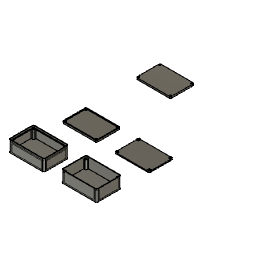
Customizable_project_box_v2_v3 (Autodesk Fusion 360 design; units mm, degrees)
Autodesk Fusion 360 part; units mm, degrees
sketch "Box footprint" plane through (0, 0, 0) normal (0, 0, 1) x (1, 0, 0)
  line L0 (0, 0) -> (130, 0)
  line L1 (130, 0) -> (130, 90)
  line L2 (130, 90) -> (0, 90)
  line L3 (0, 90) -> (0, 0)
  circle A0 centre (125.5, 85.5) radius 1.35
  line L4 (130, 90) -> (121, 90)
  line L5 (121, 90) -> (121, 81)
  line L6 (121, 81) -> (130, 81)
  line L7 (130, 81) -> (130, 90)
  line L8 (0, 81) -> (9, 81)
  line L9 (0, 90) -> (0, 81)
  line L10 (9, 81) -> (9, 90)
  line L11 (9, 90) -> (0, 90)
  circle A1 centre (4.5, 85.5) radius 1.35
  line L12 (121, 0) -> (130, 0)
  line L13 (121, 9) -> (121, 0)
  line L14 (130, 0) -> (130, 9)
  line L15 (130, 9) -> (121, 9)
  circle A2 centre (125.5, 4.5) radius 1.35
  line L16 (0, 0) -> (9, 0)
  line L17 (0, 9) -> (0, 0)
  line L18 (9, 0) -> (9, 9)
  line L19 (9, 9) -> (0, 9)
  circle A3 centre (4.5, 4.5) radius 1.35
  line L20 (4, 4) -> (126, 4) construction
  line L21 (126, 4) -> (126, 86) construction
  line L22 (126, 86) -> (4, 86) construction
  line L23 (4, 86) -> (4, 4) construction
  arc A4 (0, 4) -> (4, 0) centre (4, 4) ccw
  arc A5 (4, 90) -> (0, 86) centre (4, 86) ccw
  arc A6 (130, 86) -> (126, 90) centre (126, 86) ccw
  arc A7 (126, 0) -> (130, 4) centre (126, 4) ccw
  point P0 (125.5, 85.5)
  dimension "d1" = 130
  dimension "d2" = 90
  dimension "d13" = 2.7
  dimension "d14" = 9
  dimension "d15" = 9
  dimension "d19" = 2.7
  dimension "d20" = 9
  dimension "d21" = 9
  dimension "d22" = 2.7
  dimension "d23" = 9
  dimension "d24" = 9
  dimension "d28" = 2.7
  dimension "d29" = 9
  dimension "d30" = 9
  dimension "d125" = 4.5
  dimension "d126" = 4.5
  dimension "d127" = 4.5
  dimension "d128" = 4.5
  dimension "d177" = 4
  dimension "d178" = 4
  dimension "d179" = 4
  dimension "d180" = 4
  constraint horizontal L0
  constraint vertical L1
  constraint horizontal L2
  constraint vertical L3
  constraint coincident L0.start L3.end
  constraint horizontal L4
  constraint perpendicular L4 L5
  constraint parallel L4 L6
  constraint parallel L5 L7
  constraint coincident P0 A0.centre
  constraint horizontal L11
  constraint perpendicular L9 L11
  constraint parallel L8 L11
  constraint parallel L9 L10
  constraint horizontal L15
  constraint perpendicular L13 L15
  constraint parallel L12 L15
  constraint parallel L13 L14
  constraint horizontal L19
  constraint perpendicular L17 L19
  constraint parallel L16 L19
  constraint parallel L17 L18
  constraint coincident L2.end L3.start
  constraint coincident L0.end L1.start
  constraint vertical A1.centre A3.centre
  constraint vertical P0 A2.centre
  constraint horizontal P0 A1.centre
  constraint horizontal A2.centre A3.centre
  constraint horizontal L20
  constraint vertical L21
  constraint horizontal L22
  constraint vertical L23
  constraint coincident L17 A4.start
  constraint coincident L20.start L23.end
  constraint horizontal L20.start A4.start
  constraint vertical L20.start A4.end
  constraint coincident L9 A5.end
  constraint coincident L22.end L23.start
  constraint horizontal L22.end A5.end
  constraint vertical L22.end A5.start
  constraint coincident L4 A6.end
  constraint coincident L21.end L22.start
  constraint vertical L21.end A6.end
  constraint horizontal L21.end A6.start
  constraint coincident L12 A7.start
  constraint coincident L20.end L21.start
  constraint vertical L20.end A7.start
  constraint horizontal L20.end A7.end
  measures "d1" distance of L0.start L0.end
  measures "d2" distance of L0.start L2.end
  measures "d13" diameter of A0
  measures "d14" distance of L5.end L6.end
  measures "d15" distance of L4.end L5.end
  measures "d19" diameter of A1
  measures "d20" distance of L8.start L8.end
  measures "d21" distance of L2.end L8.start
  measures "d22" diameter of A2
  measures "d23" distance of L12.start L0.end
  measures "d24" distance of L13.start L12.start
  measures "d28" diameter of A3
  measures "d29" distance of L0.start L16.end
  measures "d30" distance of L17.start L0.start
  measures "d125" distance of A1.centre L9
  measures "d126" distance of L1 P0
  measures "d127" distance of L0 A2.centre
  measures "d128" distance of L2 P0
  measures "d177" distance of L0 L20
  measures "d178" distance of L3 L23
  measures "d179" distance of L1 L21
  measures "d180" distance of L2 L22
extrude "Extrude1" add sketch "Box footprint" against normal blind 4 contours L0 L3 L16 L17 L18 L19 A4 | L0 L1 L2 L3 L5 L6 L8 L10 L13 L15 L18 L19 | L0 L1 L12 L13 L14 L15 A7 | L2 L3 L8 L9 L10 L11 A5 | L1 L2 L4 L5 L6 L7 A6 | A0 | A1 | A2 | A3 makes body 1
extrude "Extrude5" add sketch "Box footprint" along normal blind 2 contours L0 L3 L16 L17 L18 L19 A4 | L0 L1 L12 L13 L14 L15 A7 | L2 L3 L8 L9 L10 L11 A5 | L1 L2 L4 L5 L6 L7 A6 | A0 | A1 | A2 | A3 bodies 1
sketch "Lid outline" plane through (0, 0, -4) normal (0, 0, -1) x (1, 0, 0)
  arc A0 (4, 0) -> (0, -4) centre (4, -4) ccw
  arc A1 (0, -86) -> (4, -90) centre (4, -86) ccw
  arc A2 (126, -90) -> (130, -86) centre (126, -86) ccw
  arc A3 (130, -4) -> (126, 0) centre (126, -4) ccw
  line L0 (126, 0) -> (4, 0)
  line L1 (0, -4) -> (0, -86)
  line L2 (4, -90) -> (126, -90)
  line L3 (130, -86) -> (130, -4)
  line L4 (-0.2, -4) -> (-0.2, -86)
  arc A4 (-0.2, -86) -> (4, -90.2) centre (4, -86) ccw
  line L5 (4, -90.2) -> (126, -90.2)
  arc A5 (126, -90.2) -> (130.2, -86) centre (126, -86) ccw
  line L6 (130.2, -86) -> (130.2, -4)
  arc A6 (130.2, -4) -> (126, 0.2) centre (126, -4) ccw
  line L7 (126, 0.2) -> (4, 0.2)
  arc A7 (4, 0.2) -> (-0.2, -4) centre (4, -4) ccw
  line L8 (126, 2) -> (4, 2)
  arc A8 (4, 2) -> (-2, -4) centre (4, -4) ccw
  line L9 (-2, -4) -> (-2, -86)
  arc A9 (-2, -86) -> (4, -92) centre (4, -86) ccw
  line L10 (4, -92) -> (126, -92)
  arc A10 (126, -92) -> (132, -86) centre (126, -86) ccw
  line L11 (132, -86) -> (132, -4)
  arc A11 (132, -4) -> (126, 2) centre (126, -4) ccw
  line L12 (121, -9) -> (121, 0.2)
  line L13 (121, -9) -> (130.2, -9)
  line L14 (121, -81) -> (121, -90.2)
  line L15 (121, -81) -> (130.2, -81)
  line L16 (9, -81) -> (9, -90.2)
  line L17 (9, -81) -> (-0.2, -81)
  line L18 (9, -9) -> (-0.2, -9)
  line L19 (9, -9) -> (9, 0.2)
  circle A12 centre (4.5, -85.5) radius 1.35
  circle A13 centre (4.5, -4.5) radius 1.35
  circle A14 centre (125.5, -4.5) radius 1.35
  circle A15 centre (125.5, -85.5) radius 1.35
  point P0 (9, -9)
  point P1 (9, -81)
  point P2 (121, -81)
  point P3 (121, -9)
  dimension "d181" = 0.2
  dimension "d182" = 2
  constraint coincident A3.end L0.start
  constraint coincident A0.start L0.end
  constraint coincident A0.end L1.start
  constraint coincident A1.start L1.end
  constraint coincident A1.end L2.start
  constraint coincident A2.start L2.end
  constraint coincident A2.end L3.start
  constraint coincident A3.start L3.end
  constraint coincident P3 L12.start
  constraint coincident L7 L12.end
  constraint perpendicular L7 L12
  constraint coincident L6 L13.end
  constraint perpendicular L6 L13
  constraint coincident P2 L14.start
  constraint coincident L5 L14.end
  constraint perpendicular L5 L14
  constraint coincident L6 L15.end
  constraint perpendicular L6 L15
  constraint coincident P1 L16.start
  constraint coincident L5 L16.end
  constraint perpendicular L5 L16
  constraint coincident L4 L17.end
  constraint perpendicular L4 L17
  constraint coincident P0 L18.start
  constraint coincident L4 L18.end
  constraint perpendicular L4 L18
  constraint coincident L7 L19.end
  constraint perpendicular L7 L19
extrude "Extrude8" add sketch "Lid outline" against normal blind 39 separate body contours L8 A8 L9 A9 L10 A10 L11 A11 makes body 2
sketch "Lid screw holes" plane through (0, 0, 35) normal (0, 0, 1) x (-1, 0, 0)
  circle A0 centre (-4.5, -85.5) radius 1.7
  circle A1 centre (-4.5, -4.5) radius 1.7
  circle A2 centre (-125.5, -4.5) radius 1.7
  circle A3 centre (-125.5, -85.5) radius 1.7
  circle A4 centre (-125.5, -85.5) radius 3
  circle A5 centre (-125.5, -4.5) radius 3
  circle A6 centre (-4.5, -4.5) radius 3
  circle A7 centre (-4.5, -85.5) radius 3
  arc A8 (0.2, -4) -> (-4, 0.2) centre (-4, -4) ccw
  line L0 (0.2, -4) -> (0.2, -86)
  arc A9 (-4, -90.2) -> (0.2, -86) centre (-4, -86) ccw
  line L1 (-4, -90.2) -> (-126, -90.2)
  arc A10 (-130.2, -86) -> (-126, -90.2) centre (-126, -86) ccw
  line L2 (-130.2, -86) -> (-130.2, -4)
  arc A11 (-126, 0.2) -> (-130.2, -4) centre (-126, -4) ccw
  line L3 (-126, 0.2) -> (-4, 0.2)
  arc A12 (-126, 2) -> (-132, -4) centre (-126, -4) ccw
  line L4 (-132, -4) -> (-132, -86)
  arc A13 (-132, -86) -> (-126, -92) centre (-126, -86) ccw
  line L5 (-126, -92) -> (-4, -92)
  arc A14 (-4, -92) -> (2, -86) centre (-4, -86) ccw
  line L6 (2, -86) -> (2, -4)
  arc A15 (2, -4) -> (-4, 2) centre (-4, -4) ccw
  line L7 (-4, 2) -> (-126, 2)
  point P0 (-4.5, -85.5)
  point P1 (-4.5, -4.5)
  point P2 (-125.5, -4.5)
  point P3 (-125.5, -85.5)
  point P4 (-4, -76)
  point P5 (-4, -76)
  dimension "d63" = 3.4
  dimension "d64" = 3.4
  dimension "d65" = 3.4
  dimension "d66" = 3.4
  dimension "d67" = 6
  dimension "d68" = 6
  dimension "d69" = 6
  dimension "d70" = 6
  constraint coincident P1 A1.centre
  constraint concentric A3 A4
  constraint concentric A2 A5
  constraint concentric A1 A6
  constraint concentric A0 A7
  constraint coincident P0 A0.centre
  constraint coincident P2 A2.centre
  constraint coincident P3 A3.centre
  measures "d63" diameter of A0
  measures "d64" diameter of A1
  measures "d65" diameter of A2
  measures "d66" diameter of A3
  measures "d67" diameter of A4
  measures "d68" diameter of A5
  measures "d69" diameter of A6
  measures "d70" diameter of A7
extrude "Extrude9" add sketch "Lid screw holes" along normal blind 4 contours A0 | A1 | A2 | A3 | A4 | A5 | A6 | A7 | A8 L0 A9 L1 A10 L2 A11 L3 | A12 L4 A13 L5 A14 L6 A15 L7 bodies 2
extrude "Extrude16" add sketch "Lid outline" against normal up to surface (33 mm away) from surface at -6 contours A0 L0 L1 L18 L19 | A0 L0 L1 L4 L7 A7 L18 L19 | A3 L0 L3 L6 A6 L7 L12 L13 | A3 L0 L3 L12 L13 | A1 L1 L2 L16 L17 | A1 L1 L2 L4 A4 L5 L16 L17 | A2 L2 L3 L5 A5 L6 L14 L15 | A2 L2 L3 L14 L15 | A12 | A13 | A14 | A15 bodies 2
extrude "Extrude17" cut sketch "Lid outline" against normal blind 12 from surface at -6 contours A12 | A13 | A14 | A15 bodies 2
chamfer "Chamfer3" distance 0.8 angle 45 4 edges at (3.2414, 4.0118, 2) (124.2414, 4.0118, 2) (124.2414, 85.0118, 2) (3.2414, 85.0118, 2) on bodies 2
extrude "Extrude18" cut sketch "Lid screw holes" against normal up to surface (6 mm away) from surface at -33 contours A0 | A1 | A2 | A3 bodies 1
extrude "Extrude19" cut sketch "Lid screw holes" along normal blind 4 from surface at -39 contours A4 | A5 | A6 | A7 bodies 1
extrude "Extrude20" add sketch "Lid screw holes" along normal blind 0.2 from surface at -35 contours A0 | A1 | A2 | A3 bodies 1
sketch "Lid rebate" plane through (0, 0, 35) normal (0, 0, -1) x (1, 0, 0)
  line L0 (121, -2.8) -> (9, -2.8)
  line L1 (9, -87.2) -> (121, -87.2)
  line L2 (2.8, -9) -> (2.8, -81)
  line L3 (127.2, -81) -> (127.2, -9)
  line L4 (9, -81) -> (9, -90.2)
  line L5 (9, -81) -> (-0.2, -81)
  line L6 (4, -90.2) -> (126, -90.2)
  line L7 (-0.2, -4) -> (-0.2, -86)
  line L8 (9, -9) -> (-0.2, -9)
  line L9 (9, -9) -> (9, 0.2)
  line L10 (126, 0.2) -> (4, 0.2)
  line L11 (121, -9) -> (121, 0.2)
  line L12 (121, -9) -> (130.2, -9)
  line L13 (130.2, -86) -> (130.2, -4)
  line L14 (121, -81) -> (121, -90.2)
  line L15 (121, -81) -> (130.2, -81)
  dimension "d189" = 3
  dimension "d190" = 3
  dimension "d191" = 3
  dimension "d192" = 3
  constraint coincident L0.start L11
  constraint coincident L0.end L9
  constraint coincident L2.start L8
  constraint coincident L2.end L5
  constraint coincident L1.start L4
  constraint coincident L1.end L14
  constraint coincident L3.start L15
  constraint coincident L3.end L12
  measures "d189" distance of L1 L6
  measures "d190" distance of L3 L13
  measures "d191" distance of L0 L10
  measures "d192" distance of L2 L7
sketch "Lip" plane through (0, 0, 0) normal (0, 0, 1) x (-1, 0, 0)
  line L0 (0, -9) -> (-9, -9)
  line L1 (-9, -9) -> (-9, 0)
  line L2 (-9, 0) -> (-121, 0)
  line L3 (-121, 0) -> (-121, -9)
  line L4 (-121, -9) -> (-130, -9)
  line L5 (-130, -9) -> (-130, -81)
  line L6 (-130, -81) -> (-121, -81)
  line L7 (-121, -81) -> (-121, -90)
  line L8 (-121, -90) -> (-9, -90)
  line L9 (-9, -90) -> (-9, -81)
  line L10 (-9, -81) -> (0, -81)
  line L11 (0, -81) -> (0, -9)
  line L12 (-121, -2.8) -> (-9, -2.8)
  line L13 (-2.8, -9) -> (-2.8, -81)
  line L14 (-127.2, -81) -> (-127.2, -9)
  line L15 (-9, -87.2) -> (-121, -87.2)
copy_body "CopyPasteBodies2" bodies 1 2 makes body 3 makes body 4
move_body "Move1" bodies 3 4 to x (1, 0, 0) y (0, 1, 0) z (0, 0, 1) at (200, 0, 0)
extrude "Extrude22" add sketch "Lip" against normal up to surface (2 mm away) from surface at 2 contours L0 L10 L11 L13 | L1 L2 L3 L12 | L7 L8 L9 L15 | L4 L5 L6 L14 bodies 1
extrude "Extrude23" add sketch "Lid rebate" against normal blind 4 from surface at 33 contours L0 L9 L10 L11 | L3 L12 L13 L15 | L2 L5 L7 L8 | L1 L4 L6 L14 bodies 2
chamfer "Chamfer2" distance 3 angle 45 4 edges at (65, 87.2, 6) (2.8, 45, 6) (127.2, 45, 6) (65, 2.8, 6) on bodies 2
fillet "Fillet3" radius 5 8 edges at (121, 9, 18.5) (9, 9, 18.5) (9, 81, 18.5) (121, 81, 18.5) (321, 9, 18.5) (209, 9, 18.5) (209, 81, 18.5) (321, 81, 18.5) on bodies 2 4
fillet "Fillet4" radius 5 8 edges at (121, 81, 1) (121, 9, 1) (9, 81, 1) (9, 9, 1) (209, 81, 1) (209, 9, 1) (321, 9, 1) (321, 81, 1) on bodies 1 3
move_body "Align1" bodies 4 to x (1, 0, 0) y (0, -1, 0) z (0, 0, -1) at (0, 90, 39)
move_body "Align2" bodies 2 to x (1, 0, 0) y (0, -1, 0) z (0, 0, -1) at (0, 90, 39)
move_body "Move2" bodies 4 2 to x (1, 0, 0) y (0, 1, 0) z (0, 0, 1) at (0, -200, 0)
copy_body "CopyPasteBodies3" bodies 1 makes body 5
move_body "Move3" bodies 5 to x (1, 0, 0) y (0, 1, 0) z (0, 0, 1) at (0, 200, 0)
extrude "Extrude24" add 1 faces at (46.0688, 257.7656, 0) along direction (0, 0, 1) up to surface (2 mm away) on bodies 5 bodies 5
sketch "Sketch10" plane through (0, 0, 2) normal (0, 0, 1) x (-1, 0, 0)
  line L0 (0, -286) -> (0, -204)
  line L1 (-4, -200) -> (-126, -200)
  line L2 (-130, -204) -> (-130, -286)
  line L3 (-126, -290) -> (-4, -290)
  circle A0 centre (-4.5, -204.5) radius 1.7
  circle A1 centre (-125.5, -285.5) radius 1.7
  circle A2 centre (-125.5, -204.5) radius 1.7
  circle A3 centre (-4.5, -285.5) radius 1.7
  arc A4 (0, -204) -> (-4, -200) centre (-4, -204) ccw
  arc A5 (-126, -200) -> (-130, -204) centre (-126, -204) ccw
  arc A6 (-130, -286) -> (-126, -290) centre (-126, -286) ccw
  arc A7 (-4, -290) -> (0, -286) centre (-4, -286) ccw
extrude "Extrude25" cut sketch "Sketch10" against normal up to surface (2 mm away) contours A0 | A1 | A2 | A3 bodies 5
move_body "Align3" bodies 5 to x (1, 0, 0) y (0, -1, 0) z (0, 0, -1) at (0, 571, 2)
sketch "Text layer" plane through (0, 0, -4) normal (0, 0, -1) x (1, 0, 0)
  arc A0 (0, -76) -> (4, -80) centre (4, -76) ccw
  line L0 (4, -80) -> (126, -80)
  arc A1 (126, -80) -> (130, -76) centre (126, -76) ccw
  line L1 (130, -76) -> (130, -4)
  arc A2 (130, -4) -> (126, 0) centre (126, -4) ccw
  line L2 (126, 0) -> (4, 0)
  arc A3 (4, 0) -> (0, -4) centre (4, -4) ccw
  line L3 (0, -4) -> (0, -76)
  line L4 (-1.2312, -30.121) -> (82.5266, -30.2634) construction
  line L5 (82.5266, -30.2634) -> (82.5411, -21.7478) construction
  line L6 (82.5411, -21.7478) -> (-1.2167, -21.6054) construction
  line L7 (-1.2167, -21.6054) -> (-1.2312, -30.121) construction
  circle A4 centre (4.5, -75.5) radius 3
  circle A5 centre (125.5, -75.5) radius 3
  circle A6 centre (125.5, -4.5) radius 3
  circle A7 centre (4.5, -4.5) radius 3
extrude "Extrude14" [rolled back] along distance -0.6 taper angle 0
equation "d1 = Length"
equation "d2 = Width"
equation "d13 = ScrewHoleRadius"
equation "d19 = ScrewHoleRadius"
equation "d22 = ScrewHoleRadius"
equation "d28 = ScrewHoleRadius"
equation "d31 = -Coverthickness"
equation "d40 = StudLength"
equation "d63 = ScrewClearHole"
equation "d64 = ScrewClearHole"
equation "d65 = ScrewClearHole"
equation "d66 = ScrewClearHole"
equation "d67 = ScrewHeadRadius"
equation "d68 = ScrewHeadRadius"
equation "d69 = ScrewHeadRadius"
equation "d70 = ScrewHeadRadius"
equation "d71 = Coverthickness"
equation "Width = 90 mm"
equation "Length = 130 mm"
equation "Height = 35 mm"
equation "ScrewHoleRadius = 2.7 mm" comment "2.7 for M3 screws"
equation "ScrewHeadRadius = 6 mm" comment "6mm for cap head M3 hex screws"
equation "clearance = 0.2 mm" comment "between lid and body"
equation "WallThickness = 1.8 mm"
equation "Coverthickness = 4 mm"
equation "d107 = -Coverthickness - Height"
equation "ScrewClearHole = 3.4 mm" comment "3.4 for an m3 screw"
equation "StudLength = 2 mm"
equation "d110 = -Coverthickness - StudLength"
equation "d181 = clearance"
equation "d182 = clearance + WallThickness"
named bodies: "Lid", "Main Body", "Lid without lip", "Main Body without lip", "Lid (1)", "Lid for printing face up"
